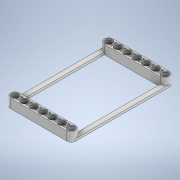
# Autodesk Inventor part: battery-adapter
Saved by Autodesk Inventor 2021 (Build 250183000, 183)
## iProperties
Created: 2024-04-09
Part Number: battery-adapter
Material: Generic
Document SubType Name: Modeling
Designer: 22hamfri
Density: 1 g/cm^3
Appearance: Default
Author: 22hamfri
Autodesk Inventor part; units mm, degrees
ref_plane "YZ Plane" through (0, 0, 0) normal (1, 0, 0) x (0, 1, 0)
ref_plane "XZ Plane" through (0, 0, 0) normal (0, 1, 0) x (-1, 0, 0)
ref_plane "XY Plane" through (0, 0, 0) normal (0, 0, 1) x (1, 0, 0)
sketch "Sketch1" plane through (0, 0, 0) normal (0, 1, 0) x (-1, 0, 0)
  line L0 (-23.71, 36.05) -> (23.71, 36.05)
  line L1 (23.71, 36.05) -> (23.71, -36.05)
  line L2 (23.71, -36.05) -> (-23.71, -36.05)
  line L3 (-23.71, -36.05) -> (-23.71, 36.05)
  line L4 (-23.71, 36.05) -> (23.71, -36.05) construction
  line L5 (23.71, 36.05) -> (-23.71, -36.05) construction
  line L6 (-27.71, 43.65) -> (27.71, 43.65)
  line L7 (27.71, 43.65) -> (27.71, -43.65)
  line L8 (27.71, -43.65) -> (-27.71, -43.65)
  line L9 (-27.71, -43.65) -> (-27.71, 43.65)
  line L10 (-27.71, 43.65) -> (27.71, -43.65) construction
  line L11 (27.71, 43.65) -> (-27.71, -43.65) construction
  circle A0 centre (23.91, 39.85) radius 3.8
  circle A1 centre (23.91, 39.85) radius 3.1
  circle A2 centre (23.91, 39.85) radius 2.575
  circle A3 centre (15.94, 39.85) radius 3.1
  circle A4 centre (15.94, 39.85) radius 2.575
  circle A5 centre (15.94, 39.85) radius 3.8
  circle A6 centre (7.97, 39.85) radius 3.1
  circle A7 centre (7.97, 39.85) radius 2.575
  circle A8 centre (7.97, 39.85) radius 3.8
  circle A9 centre (0, 39.85) radius 3.1
  circle A10 centre (0, 39.85) radius 2.575
  circle A11 centre (0, 39.85) radius 3.8
  line L12 (0, 43.65) -> (0, -43.65)
  circle A12 centre (-23.91, 39.85) radius 3.8
  circle A13 centre (-23.91, 39.85) radius 3.1
  circle A14 centre (-23.91, 39.85) radius 2.575
  circle A15 centre (-15.94, 39.85) radius 3.1
  circle A16 centre (-15.94, 39.85) radius 2.575
  circle A17 centre (-15.94, 39.85) radius 3.8
  circle A18 centre (-7.97, 39.85) radius 3.1
  circle A19 centre (-7.97, 39.85) radius 2.575
  circle A20 centre (-7.97, 39.85) radius 3.8
  line L13 (27.71, 0) -> (-27.71, 0)
  line L14 (20.8851, 37.55) -> (18.9649, 37.55)
  line L15 (12.9151, 37.55) -> (10.9949, 37.55)
  line L16 (4.9451, 37.55) -> (3.0249, 37.55)
  line L17 (-3.0249, 37.55) -> (-4.9451, 37.55)
  line L18 (-10.9949, 37.55) -> (-12.9151, 37.55)
  line L19 (-18.9649, 37.55) -> (-20.8851, 37.55)
  line L20 (20.8851, 42.15) -> (18.9649, 42.15)
  line L21 (12.9151, 42.15) -> (10.9949, 42.15)
  line L22 (4.9451, 42.15) -> (3.0249, 42.15)
  line L23 (-3.0249, 42.15) -> (-4.9451, 42.15)
  line L24 (-10.9949, 42.15) -> (-12.9151, 42.15)
  line L25 (-18.9649, 42.15) -> (-20.8851, 42.15)
  line L26 (27.71, -43.65) -> (-27.71, 43.65) construction
  circle A21 centre (23.91, -39.85) radius 3.8
  circle A22 centre (23.91, -39.85) radius 3.1
  circle A23 centre (23.91, -39.85) radius 2.575
  circle A24 centre (15.94, -39.85) radius 3.1
  circle A25 centre (15.94, -39.85) radius 2.575
  circle A26 centre (15.94, -39.85) radius 3.8
  circle A27 centre (7.97, -39.85) radius 3.1
  circle A28 centre (7.97, -39.85) radius 2.575
  circle A29 centre (7.97, -39.85) radius 3.8
  circle A30 centre (0, -39.85) radius 3.1
  circle A31 centre (0, -39.85) radius 2.575
  circle A32 centre (0, -39.85) radius 3.8
  circle A33 centre (-23.91, -39.85) radius 2.575
  circle A34 centre (-15.94, -39.85) radius 2.575
  circle A35 centre (-7.97, -39.85) radius 2.575
  circle A36 centre (-23.91, -39.85) radius 3.8
  circle A37 centre (-23.91, -39.85) radius 3.1
  circle A38 centre (-15.94, -39.85) radius 3.1
  circle A39 centre (-15.94, -39.85) radius 3.8
  circle A40 centre (-7.97, -39.85) radius 3.1
  circle A41 centre (-7.97, -39.85) radius 3.8
  line L27 (20.8851, -37.55) -> (18.9649, -37.55)
  line L28 (12.9151, -37.55) -> (10.9949, -37.55)
  line L29 (4.9451, -37.55) -> (3.0249, -37.55)
  line L30 (-3.0249, -37.55) -> (-4.9451, -37.55)
  line L31 (-10.9949, -37.55) -> (-12.9151, -37.55)
  line L32 (-18.9649, -37.55) -> (-20.8851, -37.55)
  line L33 (20.8851, -42.15) -> (18.9649, -42.15)
  line L34 (12.9151, -42.15) -> (10.9949, -42.15)
  line L35 (4.9451, -42.15) -> (3.0249, -42.15)
  line L36 (-3.0249, -42.15) -> (-4.9451, -42.15)
  line L37 (-10.9949, -42.15) -> (-12.9151, -42.15)
  line L38 (-18.9649, -42.15) -> (-20.8851, -42.15)
  line L39 (23.71, 36.05) -> (23.71, 36.0553)
  line L40 (-23.71, 36.05) -> (-23.71, 36.0553)
  line L41 (-23.71, -36.05) -> (-23.71, -36.0553)
  line L42 (23.71, -36.05) -> (23.71, -36.0553)
  point P0 (0, 0)
  point P1 (23.91, 43.65)
  point P2 (-23.91, 43.65)
  point P3 (-23.91, -43.65)
  point P4 (23.91, -43.65)
  point P5 (-27.71, 39.85)
  point P6 (-27.71, -39.85)
  point P7 (27.71, -39.85)
  point P8 (27.71, 39.85)
  dimension "d0" = 0.7
  dimension "d1" = 6.2
  dimension "d2" = 5.15
  dimension "d5" = 7.97
  dimension "d10" = 4
  dimension "d11" = 1.5
  dimension "d12" = 1.5
  dimension "d13" = 79.7
  constraints: 86 end point, 52 point on circle, 42 centre point, 34 symmetric about line, 14 collinear, 8 midpoint, 6 parallel, 6 point on line, 3 horizontal, 3 tangent, 2 perpendicular, 1 vertical, 42 other
  measures "d0" radial gap between concentric circles of A1 A0
  measures "d1" diameter of A1
  measures "d2" diameter of A2
  measures "d5" distance of A1.centre A3.centre
  measures "d10" distance between parallel lines of L7 L1
  measures "d11" distance between parallel lines of L20 L6
  measures "d12" distance between parallel lines of L0 L14
  measures "d13" distance of A30.centre A9.centre
extrude "Extrusion1" add sketch "Sketch1" along normal blind 7.76 contours L40 A12 L19 A17 L0 | A17 L18 A20 L0 | A17 | A12 | A20 L17 A11 L0 | A20 | L2 A39 L32 A36 L41 | A11 L16 A8 L0 | L12 A9 A11 | A11 L12 A9 | L25 A12 L6 A17 | L2 A41 L31 A39 | A39 | A36 | A32 L30 A41 L2 | A32 L12 A30 | L2 A29 L29 A32 | L12 A30 A32 | A8 L15 A5 L0 | A8 | L24 A17 L6 A20 | A41 | L2 A26 L28 A29 | A29 | L0 A5 L14 A0 L39 | L42 A21 L27 A26 L2 | A36 L38 A39 L8 | A5 | L23 A20 L6 A11 | A26 | A32 L8 A41 L36 | A0 | A21 | A39 L37 A41 L8 | L22 A11 L6 A8 | A29 L8 A32 L35 | A0 L20 A5 L6 | L8 A26 L33 A21 | L21 A8 L6 A5 | A26 L8 A29 L34
extrude "Extrusion2" add sketch "Sketch1" along normal blind 2 contours L3 L13 L9 A12 L40 | L3 L41 A36 L9 L13 | L13 L7 A21 L42 L1 | L1 L39 A0 L7 L13
extrude "Extrusion3" add sketch "Sketch1" along normal blind 6.96 contours L12 A10 A9 | A9 L12 A10 | A30 L12 A31 | L12 A31 A30 | A1 | A3 | A6 | A13 | A15 | A18 | A22 | A24 | A27 | A37 | A38 | A40
extrude "Extrusion4" add sketch "Sketch1" along normal blind 5.76 contours L19 A12 L25 A17 | A17 L24 A20 L18 | A20 L23 A11 L17 | A11 L22 A8 L16 | L31 A41 L37 A39 | A39 L38 A36 L32 | L29 A29 L35 A32 | A32 L36 A41 L30 | A8 L21 A5 L15 | L28 A26 L34 A29 | A5 L20 A0 L14 | L27 A21 L33 A26
sketch "Sketch2" plane through (0, 0, 0) normal (0, -1, 0) x (1, 0, 0)
  line L0 (23.71, -36.05) -> (23.71, -36.0553) projected
  arc A0 (23.91, -43.65) -> (23.71, -36.0553) centre (23.91, -39.85) ccw projected
  line L1 (23.91, -43.65) -> (-23.91, -43.65) projected
  arc A1 (-23.71, -36.0553) -> (-23.91, -43.65) centre (-23.91, -39.85) ccw projected
  line L2 (-23.71, -36.0553) -> (-23.71, -36.05) projected
  line L3 (-23.71, -36.05) -> (23.71, -36.05) projected
  arc A2 (18.9649, -42.15) -> (18.9649, -37.55) centre (15.94, -39.85) ccw projected
  line L4 (18.9649, -42.15) -> (20.8851, -42.15) projected
  arc A3 (20.8851, -37.55) -> (20.8851, -42.15) centre (23.91, -39.85) ccw projected
  line L5 (20.8851, -37.55) -> (18.9649, -37.55) projected
  arc A4 (4.9451, -37.55) -> (4.9451, -42.15) centre (7.97, -39.85) ccw projected
  line L6 (4.9451, -37.55) -> (3.0249, -37.55) projected
  arc A5 (3.0249, -42.15) -> (3.0249, -37.55) centre (0, -39.85) ccw projected
  line L7 (3.0249, -42.15) -> (4.9451, -42.15) projected
  circle A6 centre (0, -39.85) radius 3.1 projected
  line L8 (-3.0249, -37.55) -> (-4.9451, -37.55) projected
  arc A7 (-4.9451, -42.15) -> (-4.9451, -37.55) centre (-7.97, -39.85) ccw projected
  line L9 (-4.9451, -42.15) -> (-3.0249, -42.15) projected
  arc A8 (-3.0249, -37.55) -> (-3.0249, -42.15) centre (0, -39.85) ccw projected
  line L10 (-10.9949, -37.55) -> (-12.9151, -37.55) projected
  arc A9 (-12.9151, -42.15) -> (-12.9151, -37.55) centre (-15.94, -39.85) ccw projected
  line L11 (-12.9151, -42.15) -> (-10.9949, -42.15) projected
  arc A10 (-10.9949, -37.55) -> (-10.9949, -42.15) centre (-7.97, -39.85) ccw projected
  circle A11 centre (-7.97, -39.85) radius 3.1 projected
  circle A12 centre (-15.94, -39.85) radius 3.1 projected
  circle A13 centre (-23.91, -39.85) radius 3.1 projected
  arc A14 (-18.9649, -37.55) -> (-18.9649, -42.15) centre (-15.94, -39.85) ccw projected
  line L12 (-18.9649, -37.55) -> (-20.8851, -37.55) projected
  arc A15 (-20.8851, -42.15) -> (-20.8851, -37.55) centre (-23.91, -39.85) ccw projected
  line L13 (-20.8851, -42.15) -> (-18.9649, -42.15) projected
  circle A16 centre (7.97, -39.85) radius 3.1 projected
  circle A17 centre (15.94, -39.85) radius 3.1 projected
  line L14 (12.9151, -37.55) -> (10.9949, -37.55) projected
  arc A18 (10.9949, -42.15) -> (10.9949, -37.55) centre (7.97, -39.85) ccw projected
  line L15 (10.9949, -42.15) -> (12.9151, -42.15) projected
  arc A19 (12.9151, -37.55) -> (12.9151, -42.15) centre (15.94, -39.85) ccw projected
  circle A20 centre (23.91, -39.85) radius 3.1 projected
  circle A21 centre (7.97, -39.85) radius 3.1 projected
  circle A22 centre (7.97, -39.85) radius 2.575 projected
  circle A23 centre (15.94, -39.85) radius 3.1 projected
  circle A24 centre (15.94, -39.85) radius 2.575 projected
  circle A25 centre (23.91, -39.85) radius 3.1 projected
  circle A26 centre (23.91, -39.85) radius 2.575 projected
  circle A27 centre (0, -39.85) radius 3.1 projected
  circle A28 centre (0, -39.85) radius 2.575 projected
  circle A29 centre (-7.97, -39.85) radius 3.1 projected
  circle A30 centre (-7.97, -39.85) radius 2.575 projected
  circle A31 centre (-15.94, -39.85) radius 3.1 projected
  circle A32 centre (-15.94, -39.85) radius 2.575 projected
  circle A33 centre (-23.91, -39.85) radius 3.1 projected
  circle A34 centre (-23.91, -39.85) radius 2.575 projected
  circle A35 centre (-23.91, 39.85) radius 3.1 projected
  circle A36 centre (-23.91, 39.85) radius 2.575 projected
  circle A37 centre (-15.94, 39.85) radius 3.1 projected
  circle A38 centre (-15.94, 39.85) radius 2.575 projected
  circle A39 centre (-7.97, 39.85) radius 3.1 projected
  circle A40 centre (-7.97, 39.85) radius 2.575 projected
  circle A41 centre (0, 39.85) radius 3.1 projected
  circle A42 centre (0, 39.85) radius 2.575 projected
  circle A43 centre (7.97, 39.85) radius 3.1 projected
  circle A44 centre (7.97, 39.85) radius 2.575 projected
  circle A45 centre (15.94, 39.85) radius 3.1 projected
  circle A46 centre (15.94, 39.85) radius 2.575 projected
  circle A47 centre (23.91, 39.85) radius 3.1 projected
  circle A48 centre (23.91, 39.85) radius 2.575 projected
  line L16 (-23.71, 36.05) -> (-23.71, 36.0553) projected
  arc A49 (-23.91, 43.65) -> (-23.71, 36.0553) centre (-23.91, 39.85) ccw projected
  line L17 (-23.91, 43.65) -> (23.91, 43.65) projected
  arc A50 (23.71, 36.0553) -> (23.91, 43.65) centre (23.91, 39.85) ccw projected
  line L18 (23.71, 36.0553) -> (23.71, 36.05) projected
  line L19 (23.71, 36.05) -> (-23.71, 36.05) projected
  line L20 (-12.9151, 37.55) -> (-10.9949, 37.55) projected
  arc A51 (-10.9949, 42.15) -> (-10.9949, 37.55) centre (-7.97, 39.85) ccw projected
  line L21 (-10.9949, 42.15) -> (-12.9151, 42.15) projected
  arc A52 (-12.9151, 37.55) -> (-12.9151, 42.15) centre (-15.94, 39.85) ccw projected
  line L22 (-4.9451, 37.55) -> (-3.0249, 37.55) projected
  arc A53 (-3.0249, 42.15) -> (-3.0249, 37.55) centre (0, 39.85) ccw projected
  line L23 (-3.0249, 42.15) -> (-4.9451, 42.15) projected
  arc A54 (-4.9451, 37.55) -> (-4.9451, 42.15) centre (-7.97, 39.85) ccw projected
  line L24 (20.8851, 42.15) -> (18.9649, 42.15) projected
  arc A55 (18.9649, 37.55) -> (18.9649, 42.15) centre (15.94, 39.85) ccw projected
  line L25 (18.9649, 37.55) -> (20.8851, 37.55) projected
  arc A56 (20.8851, 42.15) -> (20.8851, 37.55) centre (23.91, 39.85) ccw projected
  circle A57 centre (15.94, 39.85) radius 3.1 projected
  circle A58 centre (23.91, 39.85) radius 3.1 projected
  circle A59 centre (0, 39.85) radius 3.1 projected
  circle A60 centre (7.97, 39.85) radius 3.1 projected
  line L26 (10.9949, 37.55) -> (12.9151, 37.55) projected
  arc A61 (12.9151, 42.15) -> (12.9151, 37.55) centre (15.94, 39.85) ccw projected
  line L27 (12.9151, 42.15) -> (10.9949, 42.15) projected
  arc A62 (10.9949, 37.55) -> (10.9949, 42.15) centre (7.97, 39.85) ccw projected
  line L28 (3.0249, 37.55) -> (4.9451, 37.55) projected
  arc A63 (4.9451, 42.15) -> (4.9451, 37.55) centre (7.97, 39.85) ccw projected
  line L29 (4.9451, 42.15) -> (3.0249, 42.15) projected
  arc A64 (3.0249, 37.55) -> (3.0249, 42.15) centre (0, 39.85) ccw projected
  arc A65 (-18.9649, 42.15) -> (-18.9649, 37.55) centre (-15.94, 39.85) ccw projected
  line L30 (-18.9649, 42.15) -> (-20.8851, 42.15) projected
  arc A66 (-20.8851, 37.55) -> (-20.8851, 42.15) centre (-23.91, 39.85) ccw projected
  line L31 (-20.8851, 37.55) -> (-18.9649, 37.55) projected
  circle A67 centre (-7.97, 39.85) radius 3.1 projected
  circle A68 centre (-15.94, 39.85) radius 3.1 projected
  circle A69 centre (-23.91, 39.85) radius 3.1 projected
  point P0 (0, 0)
extrude "Extrusion5" cut sketch "Sketch2" against normal blind 0.8 contours A6 | A11 | A12 | A13 | A16 | A17 | A20 | A35 | A37 | A39 | A41 | A43 | A45 | A47
extrude "Extrusion6" cut sketch "Sketch2" against normal blind 2 contours A2 L5 A3 L4 | A4 L7 A5 L6 | A8 L9 A7 L8 | A10 L11 A9 L10 | A14 L13 A15 L12 | A19 L15 A18 L14 | A52 L21 A51 L20 | A54 L23 A53 L22 | A56 L25 A55 L24 | A62 L27 A61 L26 | A64 L29 A63 L28 | A65 L31 A66 L30
body "Solid1"
